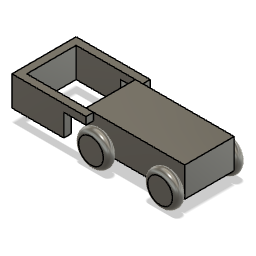
Prototype3_v2 v0 (Autodesk Fusion 360 design; units mm, degrees)
Autodesk Fusion 360 part; units mm, degrees
sketch "Sketch1" plane through (0, 0, 0) normal (0, 1, 0) x (1, 0, 0)
  line L0 (0, 5) -> (20, 5)
  line L1 (20, 5) -> (20, -5)
  line L2 (20, -5) -> (0, -5)
  line L3 (0, -5) -> (0, 5)
  line L4 (0, 0) -> (20, 0) construction
  dimension "d33" = 10
  dimension "d34" = 20
  constraint horizontal L0
  constraint vertical L1
  constraint horizontal L2
  constraint vertical L3
  constraint coincident L4.start L3
  constraint midpoint L3 L4.start
  constraint midpoint L1 L4.end
  constraint coincident origin L4
  measures "d33" distance of L0.end L1.end
  measures "d34" distance of L0.start L0.end
extrude "Extrude1" add sketch "Sketch1" along normal blind 6 makes body 1
sketch "Sketch3" plane through (0, 0, 5) normal (0, 0, 1) x (1, 0, 0)
  line L0 (0, 0) -> (20, 0)
  line L1 (20, 0) -> (20, 6) construction
  line L2 (20, 6) -> (0, 6)
  line L3 (0, 6) -> (0, 0)
  circle A0 centre (3, 1) radius 3.5
  line L4 (10, 6) -> (10, 0) construction
  circle A1 centre (17, 1) radius 3.5
  line L5 (20, 3) -> (0, 3) construction
  dimension "d5" = 7
  dimension "d6" = 3
  dimension "d35" = 2
  constraint midpoint L2 L4.start
  constraint midpoint L0 L4.end
  constraint symmetric A0 L4 A1
  constraint midpoint L1 L5.start
  constraint midpoint L3 L5.end
  measures "d5" diameter of A1
  measures "d6" distance of L1 A1.centre
  measures "d35" distance of A1.centre L5
extrude "Extrude3" add sketch "Sketch3" along normal blind 2 separate body makes body 2 at (20.4826, 0.6515, 5.6667) makes body 3 at (6.4826, 1.3485, 6.3333)
fillet "Fillet1" radius 1 1 edges at (-0.2631, -0.2657, 5) 4 faces at (3.9577, 1.1135, 5) (3.5084, 1.7675, 7) (19.2048, 0.3199, 7) (16.2726, 0.0879, 5) on bodies 2 3
mirror "Mirror1" about plane through (0, 0, 0) normal (0, 0, 1) of bodies 2 3 makes body 4 at (6.4646, 0.6533, -5.8106) makes body 5 at (20.4646, 0.6533, -5.8106)
copy_body "Body->Comp1" bodies 1 removing the originals makes body 6 in component "Component"
copy_body "Body->Comp2" bodies 3 removing the originals makes body 7 in component "Component'"
copy_body "Body->Comp3" bodies 2 removing the originals makes body 8 in component "Component''"
copy_body "Body->Comp4" bodies 4 removing the originals makes body 9 in component "Component'''"
copy_body "Body->Comp5" bodies 5 removing the originals makes body 10 in component "Component''''"
sketch "Sketch5" plane through (0, 0, 0) normal (0, 1, 0) x (1, 0, 0)
  line L0 (-13.5, 6.5) -> (1.5, 6.5)
  line L1 (1.5, 6.5) -> (1.5, -6.5)
  line L2 (1.5, -6.5) -> (-13.5, -6.5)
  line L3 (-13.5, -6.5) -> (-13.5, 6.5)
  line L4 (0, -5) -> (-12, -5)
  line L5 (-12, -5) -> (-12, 5)
  line L6 (-12, 5) -> (0, 5)
  line L7 (0, 5) -> (0, -5)
  line L8 (0, 5) -> (0, -5) construction
  line L9 (0, 0) -> (-12, 0) construction
  dimension "d18" = 1.5
  dimension "d36" = 13
  dimension "d39" = 15
  constraint horizontal L0
  constraint vertical L1
  constraint horizontal L2
  constraint vertical L3
  constraint midpoint L7 L9.start
  constraint midpoint L5 L9.end
  constraint coincident origin L9
  constraint collinear L7 L8
  measures "d36" distance of L0.start L2.end
  measures "d39" distance of L1 L3
extrude "Extrude1'" add sketch "Sketch5" along normal blind 6 separate body makes body 11 in component "Component'''''"
sketch "Sketch7" plane through (0, 0, 6.5) normal (0, 0, 1) x (1, 0, 0)
  line L0 (-13.5, 0) -> (1.5, 0)
  line L1 (1.5, 0) -> (1.5, 6)
  line L2 (1.5, 6) -> (-13.5, 6)
  line L3 (-13.5, 6) -> (-13.5, 0)
  circle A0 centre (0.5, 1) radius 0.75
  dimension "d23" = 1.5
  dimension "d24" = 1
  measures "d23" diameter of A0
  measures "d24" distance of L1 A0.centre
sketch "Sketch9" plane through (0, 0, 6.5) normal (0, 0, 1) x (1, 0, 0)
  line L0 (-13.5, 0) -> (1.5, 0)
  line L1 (1.5, 0) -> (1.5, 6)
  line L2 (1.5, 6) -> (-13.5, 6)
  line L3 (-13.5, 6) -> (-13.5, 0)
  line L4 (-3, 4.5) -> (1.5, 4.5)
  line L5 (1.5, 4.5) -> (1.5, 0)
  line L6 (1.5, 0) -> (-3, 0)
  line L7 (-3, 0) -> (-3, 4.5)
  dimension "d44" = 1.5
  constraint horizontal L4
  constraint vertical L5
  constraint horizontal L6
  constraint vertical L7
  constraint coincident L0.end L1.start
  constraint equal L4 L7
  measures "d44" distance of L2 L4
extrude "Extrude2" [suppressed] in component "Component"
extrude "Extrude1''" [no effect] in component "Component'"
extrude "Extrude1'''" [no effect] in component "Component'''"
extrude "Extrude4" cut sketch "Sketch9" against normal through all contours L0 L1 L4 L5 L6 L7 bodies 11 in component "Component'''''"
sketch "Sketch10" plane through (0, 6, 0) normal (0, 1, 0) x (-1, 0, 0)
  line L0 (12, -5) -> (0, -5)
  line L1 (0, -5) -> (0, 5)
  line L2 (0, 5) -> (12, 5)
  line L3 (12, 5) -> (12, -5)
  line L4 (13.5, 6.5) -> (-1.5, 6.5)
  line L5 (-1.5, 6.5) -> (-1.5, -6.5)
  line L6 (-1.5, -6.5) -> (13.5, -6.5)
  line L7 (13.5, -6.5) -> (13.5, 6.5)
  line L8 (0, -5) -> (-1.5, -5)
  line L9 (-1.5, -5) -> (-1.5, 5)
  line L10 (-1.5, 5) -> (0, 5)
  line L11 (0, 5) -> (0, -5)
  dimension "d45" = 10
  constraint horizontal L8
  constraint vertical L9
  constraint horizontal L10
  constraint vertical L11
  constraint coincident L0.end L1.start
  measures "d45" distance of L0.end L1.end
extrude "Extrude5" cut sketch "Sketch10" against normal blind 1.5 contours L1 L5 L8 L9 L10 L11 bodies 11 in component "Component'''''"
component "Component" placed x (1, 0, 0) y (0, 1, 0) z (0, 0, 1) at (0, 0, 0)
component "Component'" placed x (1, 0, 0) y (0, 1, 0) z (0, 0, 1) at (0, 0, 0)
component "Component''" placed x (1, 0, 0) y (0, 1, 0) z (0, 0, 1) at (0, 0, 0)
component "Component'''" placed x (1, 0, 0) y (0, 1, 0) z (0, 0, 1) at (0, 0, 0)
component "Component''''" placed x (1, 0, 0) y (0, 1, 0) z (0, 0, 1) at (0, 0, 0)
component "Component'''''" placed x (1, 0, 0) y (0, 1, 0) z (0, 0, 1) at (0, 0, 0)
